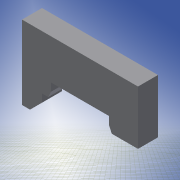
# Autodesk Inventor part: _WT_Aufnahme_Antriebseinheit3
Saved by Autodesk Inventor 2019 (Build 230136000, 136)
## iProperties
Created: 2025-05-01
Part Number: _WT_Aufnahme_Antriebseinheit3
Material: Generisch
Document SubType Name: Modeling
Designer: RP
Density: 1 g/cm^3
Appearance: Vorgabe
Author: RP
Autodesk Inventor part; units mm, degrees
ref_plane "YZ Plane" through (0, 0, 0) normal (1, 0, 0) x (0, 1, 0)
ref_plane "XZ Plane" through (0, 0, 0) normal (0, 1, 0) x (-1, 0, 0)
ref_plane "XY Plane" through (0, 0, 0) normal (0, 0, 1) x (1, 0, 0)
sketch "Skizze1" plane through (0, 0, 0) normal (0, 0, 1) x (1, 0, 0)
  line L0 (-19, -11) -> (-19, -7)
  line L1 (-19, -7) -> (-15.8989, -7)
  line L2 (-15.8989, -7) -> (-14.5, -4)
  line L3 (-14.5, -4) -> (-14.5, 0)
  line L4 (-14.5, 0) -> (14.5, 0)
  line L5 (14.5, 0) -> (14.5, -4)
  line L6 (14.5, -4) -> (15.8989, -7)
  line L7 (15.8989, -7) -> (19, -7)
  line L8 (19, -7) -> (19, -11)
  line L9 (19, -11) -> (25, -17)
  line L10 (25, -17) -> (29, -17)
  line L11 (29, -17) -> (29, 20)
  line L12 (29, 20) -> (-29, 20)
  line L13 (-29, 20) -> (-29, -17)
  line L14 (-29, -17) -> (-25, -17)
  line L15 (-25, -17) -> (-19, -11)
  line L16 (0, 0) -> (0, -29.3821)
  dimension "d5" = 29
  dimension "d6" = 20
  dimension "d7" = 4
  dimension "d8" = 4.5
  dimension "d10" = 38
  dimension "d12" = 25
  dimension "d13" = 10
  dimension "d14" = 10
  dimension "d15" = 7
  dimension "d16" = 45
  dimension "d17" = 10
  dimension "d18" = 4
  constraints: 35 end point, 9 perpendicular, 3 parallel, 2 point on line, 2 vertical, 1 collinear, 1 midpoint, 2 other
  measures "d5" distance of L3.end L4.end
  measures "d6" distance between parallel lines of L12 L4
  measures "d7" distance of L2.end L3.end
  measures "d8" distance between parallel lines of L3 L0
  measures "d10" distance between parallel lines of L0 L8
  measures "d12" angle of L2 L3
  measures "d13" distance between parallel lines of L0 L13
  measures "d14" distance between parallel lines of L11 L8
  measures "d15" distance between parallel lines of L1 L4
  measures "d16" angle of L0 L15
  measures "d17" distance between parallel lines of L1 L14
  measures "d18" distance of L0.start L0.end
extrude "Extrusion1" add sketch "Skizze1" along normal mid plane 10
sketch "Skizze2" plane through (25, -17, 5) normal (0, -1, 0) x (1, 0, 0)
  line L0 (4, -10) -> (4, 0) projected
  line L1 (-54, -10) -> (4, -10) projected
  line L2 (4, 0) -> (-6, 0)
  line L3 (-6, 0) -> (-6, -10)
  line L4 (-6, -10) -> (4, -10)
  line L5 (4, -10) -> (4, 0)
  point P0 (-25, -5)
  dimension "d21" = 10
  constraints: 8 end point, 2 parallel, 1 horizontal, 1 perpendicular, 1 point on line
  measures "d21" distance of L0.end L2.end
extrude "Extrusion2" cut sketch "Skizze2" against normal blind 10
